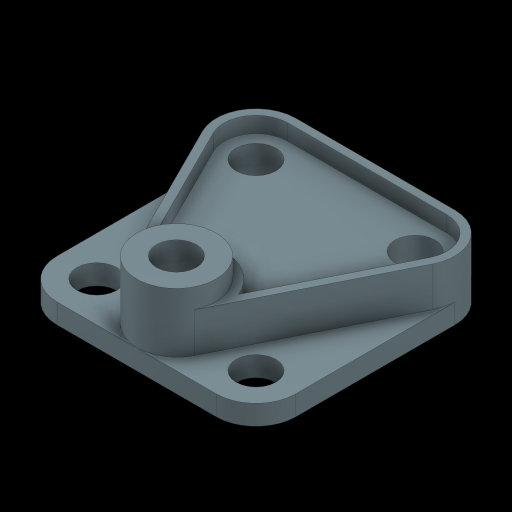
# Autodesk Inventor part: ANS12-6-BK
Saved by Autodesk Inventor 2024 (Build 280153000, 153)
## iProperties
Created: 2023-12-13
Part Number: ANS12-6-BK
Material: Lead
Document SubType Name: Modeling
Designer: bennk
Mass: 749.217 g
Surface Area: 192.235 cm^2
Volume: 66.0686 cm^3
Density: 11.34 g/cm^3
Appearance: Lead
Author: bennk
Autodesk Inventor part; units mm, degrees
ref_plane "YZ Plane" through (0, 0, 0) normal (1, 0, 0) x (0, 1, 0)
ref_plane "XZ Plane" through (0, 0, 0) normal (0, 1, 0) x (-1, 0, 0)
ref_plane "XY Plane" through (0, 0, 0) normal (0, 0, 1) x (1, 0, 0)
sketch "Sketch1" plane through (0, 0, 0) normal (0, 1, 0) x (-1, 0, 0)
  circle A0 centre (0, 0) radius 12.7
  circle A1 centre (0, 0) radius 6.35
  line L0 (25.4, 12.7) -> (-25.4, 12.7)
  line L1 (-38.1, 0) -> (-38.1, -50.8)
  line L2 (-25.4, -63.5) -> (25.4, -63.5)
  line L3 (38.1, -50.8) -> (38.1, 0)
  arc A2 (38.1, 0) -> (25.4, 12.7) centre (25.4, 0) ccw
  arc A3 (25.4, -63.5) -> (38.1, -50.8) centre (25.4, -50.8) ccw
  arc A4 (-38.1, -50.8) -> (-25.4, -63.5) centre (-25.4, -50.8) ccw
  arc A5 (-25.4, 12.7) -> (-38.1, 0) centre (-25.4, 0) ccw
  circle A6 centre (25.4, 0) radius 6.35
  circle A7 centre (25.4, -50.8) radius 6.35
  circle A8 centre (-25.4, -50.8) radius 6.35
  circle A9 centre (-25.4, 0) radius 6.35
  arc A10 (25.4, -63.5) -> (36.7592, -45.1204) centre (25.4, -50.8) ccw
  line L4 (11.3592, 5.6796) -> (36.7592, -45.1204)
  line L5 (14.1674, -5.6163) -> (34.4874, -46.2563)
  arc A11 (-15.1267, -1.8552) -> (14.1674, -5.6163) centre (0, 0) ccw
  circle A12 centre (25.4, -50.8) radius 10.16
  line L6 (25.4, -60.96) -> (0, -60.96)
  line L7 (0, 0) -> (0, -63.5)
  line L8 (-11.3592, 5.6796) -> (-36.7592, -45.1204)
  line L9 (-14.1674, -5.6163) -> (-34.4874, -46.2563)
  circle A13 centre (-25.4, -50.8) radius 10.16
  line L10 (-25.4, -60.96) -> (0, -60.96)
  arc A14 (-36.7592, -45.1204) -> (-25.4, -63.5) centre (-25.4, -50.8) ccw
  point P0 (-34.4874, -46.2563)
  dimension "d0" = 25.4
  dimension "d1" = 12.7
  dimension "d2" = 63.5
  dimension "d3" = 76.2
  dimension "d4" = 38.1
  dimension "d5" = 12.7
  dimension "d6" = 12.7
  dimension "d7" = 2.54
  dimension "d8" = 2.54
  dimension "d9" = 2.54
  dimension "d10" = 25.4
  dimension "d11" = 3.6126
  constraints: 22 end point, 15 point on circle, 12 centre point, 8 coincident, 7 tangent, 6 equal radius, 6 symmetric about line, 3 parallel, 3 point on line, 2 horizontal, 2 perpendicular, 1 midpoint, 1 vertical, 10 other
  measures "d1" diameter of A1
  measures "d2" distance from line of point (0, 0) L2
  measures "d3" distance between parallel lines of L3 L1
  measures "d4" distance from line of point (0, 0) L3
  measures "d5" radius of A2
  measures "d6" diameter of A6
  measures "d7" distance between parallel lines of L4 L5
  measures "d10" distance of L6.start L6.end
  measures "d11" distance from line of L5.end L3
extrude "BASE" add sketch "Sketch1" against normal blind 6.35
extrude "RAISED FLOOR" add sketch "Sketch1" along normal blind 7.62 contours L7 L10 A13 L9 A11 | A11 L5 A12 L6 L7 | A13 | A12
extrude "EDGE" add sketch "Sketch1" along normal blind 12.7 contours A0 L4 A10 A3 L2 L7 L6 A12 L5 A11 | L7 A11 L8 A0 | A11 L9 A13 L10 L7 L2 A4 A14 L8
extrude "COLLUMN" add sketch "Sketch1" along normal blind 19.05 contours A0
equation "\"d4\" = 0.5 * d3"
body "Solid1"
